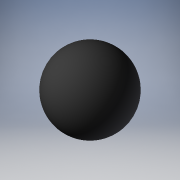
# Autodesk Inventor part: 51200 Ball
Saved by Autodesk Inventor 2019 (Build 230136000, 136)
## iProperties
Created: 2023-01-10
Part Number: 51200 Ball
Material: Generic
Catalog Web Link: www.cadenas.de
Description: With flat seet B-
Vendor: NSK_RB
Document SubType Name: Modeling
Designer: psAdmin
Manufacturer: NSK_RB
Mass: 0.0871137 g
Surface Area: 0.950332 cm^2
Volume: 0.0871137 cm^3
Density: 1 g/cm^3
Appearance: PSOLRGB-175-175-175
Category: PARTsolutions
Company: NSK_RB
Title: 51200 Ball
Author: Cadenas PARTsolutions
PSOL_IDENT_0: {$CADENAS_DATA/23d-libs/nsk_rb/roller_bearings/thrust_bearings/single_direction_tbb/with_flat_seet_b
PSOL_IDENT_1: .prj},172 {VTYP=3D},{NB=51200 Ball},{LINA=51200 Ball},{NN=With flat seet B},{DATE=27.09.2022 23:23:1
PSOL_IDENT_2: 0},{GEOMDATE=02.08.2010 09:29:00},{VERSION=},{LINEID=6260},{WBVAR=},{WBNUMERIC=}  {NB=51200 Ball},{L
PSOL_IDENT_3: INA=51200 Ball},{KT=DUMMY},{IDNR=},{STAN=},{NO=2},{ORDER=51200},{SD=10},{D=26},{T=11},{T3=11.6},{T4=
PSOL_IDENT_4: 13},{SR=0.6},{CAN=12800},{COAN=17100},{CA=1300},{COA=1740},{GRE=6000},{OIL=9000},{SD1=26},{D1=12},{D
PSOL_IDENT_5: 2=18},{D3=28},{SB=3.5},{A=8.5},{R=22},{SDA=20},{DA=16},{SRA=0.6},{MASS=0.028},{N=10}
NB: 51200 Ball
NN: With flat seet B
NBSYN: $ORDER. Ball
LINA: 51200 Ball
CATALOG: NSK Rolling Bearing
NO: 2
ORDER: 51200
SD: 10
D: 26
T: 11
T3: 11.6
T4: 13
SR: 0.6
CAN: 12800
COAN: 17100
CA: 1300
COA: 1740
GRE: 6000
OIL: 9000
SD1: 26
D1: 12
D2: 18
D3: 28
SB: 3.5
A: 8.5
R: 22
SDA: 20
DA: 16
SRA: 0.6
MASS: 0.028
N: 10
SUPPLIER: NSK_RB
ARTICLENO: 51200 Ball
BOMINFO: 51200 Ball
CREATOR: CADENAS GmbH
Autodesk Inventor part; units mm, degrees
sketch "Sketch_1" plane through (0, 0, 0) normal (0, 0, 1) x (1, 0, 0)
  line L0 (2.75, 0) -> (-2.75, 0)
  arc A0 (2.75, 0) -> (-2.75, 0) centre (0, 0) ccw
  line L1 (2.75, 0) -> (-2.75, 0)
  constraints: 4 end point, 2 point on circle, 1 centre point
revolve "Revolution1" add sketch "Sketch_1" angle 360 about axis through (2.75, 0, 0) along (1, 0, 0)
ref_plane "B_HW_XY" through (0, 0, 0) normal (1, 0, 0) x (0, 0, -1)
ref_plane "B_HW_YZ" through (0, 0, 0) normal (0, 0, -1) x (0, 1, 0)
ref_plane "B_HW_ZX" through (0, 0, 0) normal (0, 1, 0) x (1, 0, 0)
body "Solid1"
